Autodesk Inventor part; units mm, degrees
(part 2 of 3)
  circle A470 centre (-52.8488, 38.1375) radius 0.851
  circle A471 centre (-42.6888, 38.1375) radius 0.851
  circle A472 centre (-38.2437, 19.0875) radius 1.994
  circle A473 centre (-43.3237, 19.0875) radius 0.851
  circle A474 centre (-33.1638, 19.0875) radius 0.851
  circle A475 centre (-33.4813, 0.0375) radius 1.994
  circle A476 centre (-38.5613, 0.0375) radius 0.851
  circle A477 centre (-28.4013, 0.0375) radius 0.851
  circle A478 centre (-23.9563, -19.0125) radius 1.994
  circle A479 centre (-29.0362, -19.0125) radius 0.851
  circle A480 centre (-18.8762, -19.0125) radius 0.851
  circle A481 centre (-135.875, 0.0375) radius 1.994
  circle A482 centre (-140.955, 0.0375) radius 0.851
  circle A483 centre (-130.795, 0.0375) radius 0.851
  circle A484 centre (-28.7188, 38.1375) radius 1.994
  circle A485 centre (-33.7987, 38.1375) radius 0.851
  circle A486 centre (-23.6388, 38.1375) radius 0.851
  circle A487 centre (-19.1938, 19.0875) radius 1.994
  circle A488 centre (-24.2737, 19.0875) radius 0.851
  circle A489 centre (-14.1137, 19.0875) radius 0.851
  circle A490 centre (-14.4313, 0.0375) radius 1.994
  circle A491 centre (-19.5113, 0.0375) radius 0.851
  circle A492 centre (-9.3513, 0.0375) radius 0.851
  circle A493 centre (-4.9062, -19.0125) radius 1.994
  circle A494 centre (-9.9863, -19.0125) radius 0.851
  circle A495 centre (0.1737, -19.0125) radius 0.851
  circle A496 centre (-21.575, -38.0625) radius 1.994
  circle A497 centre (-26.655, -38.0625) radius 0.851
  circle A498 centre (-16.495, -38.0625) radius 0.851
  circle A499 centre (-71.613, -31.0775) radius 1.524
  circle A500 centre (28.463, -31.0775) radius 1.524
  circle A501 centre (-71.613, -46.3175) radius 1.994
  circle A502 centre (28.463, -46.3175) radius 1.994
  circle A503 centre (-9.6687, 38.1375) radius 1.994
  circle A504 centre (-14.7487, 38.1375) radius 0.851
  circle A505 centre (-4.5888, 38.1375) radius 0.851
  circle A506 centre (-0.1437, 19.0875) radius 1.994
  circle A507 centre (-5.2238, 19.0875) radius 0.851
  circle A508 centre (4.9363, 19.0875) radius 0.851
  circle A509 centre (4.6188, 0.0375) radius 1.994
  circle A510 centre (-0.4612, 0.0375) radius 0.851
  circle A511 centre (9.6988, 0.0375) radius 0.851
  circle A512 centre (14.1438, -19.0125) radius 1.994
  circle A513 centre (9.0638, -19.0125) radius 0.851
  circle A514 centre (19.2237, -19.0125) radius 0.851
  circle A515 centre (-131.1125, -19.0125) radius 1.994
  circle A516 centre (-136.1925, -19.0125) radius 0.851
  circle A517 centre (-126.0325, -19.0125) radius 0.851
  circle A518 centre (-143.0505, -12.0275) radius 1.524
  circle A519 centre (-119.1745, -12.0275) radius 1.524
  circle A520 centre (-143.0505, -27.2675) radius 1.994
  circle A521 centre (-119.1745, -27.2675) radius 1.994
  circle A522 centre (9.3812, 38.1375) radius 1.994
  circle A523 centre (4.3012, 38.1375) radius 0.851
  circle A524 centre (14.4613, 38.1375) radius 0.851
  circle A525 centre (18.9062, 19.0875) radius 1.994
  circle A526 centre (13.8262, 19.0875) radius 0.851
  circle A527 centre (23.9862, 19.0875) radius 0.851
  circle A528 centre (23.6687, 0.0375) radius 1.994
  circle A529 centre (18.5888, 0.0375) radius 0.851
  circle A530 centre (28.7488, 0.0375) radius 0.851
  circle A531 centre (33.1938, -19.0125) radius 1.994
  circle A532 centre (28.1137, -19.0125) radius 0.851
  circle A533 centre (38.2737, -19.0125) radius 0.851
  circle A534 centre (28.4313, 38.1375) radius 1.994
  circle A535 centre (23.3513, 38.1375) radius 0.851
  circle A536 centre (33.5112, 38.1375) radius 0.851
  circle A537 centre (37.9562, 19.0875) radius 1.994
  circle A538 centre (32.8762, 19.0875) radius 0.851
  circle A539 centre (43.0363, 19.0875) radius 0.851
  circle A540 centre (42.7188, 0.0375) radius 1.994
  circle A541 centre (37.6388, 0.0375) radius 0.851
  circle A542 centre (47.7987, 0.0375) radius 0.851
  circle A543 centre (52.2438, -19.0125) radius 1.994
  circle A544 centre (47.1638, -19.0125) radius 0.851
  circle A545 centre (57.3238, -19.0125) radius 0.851
  circle A546 centre (-140.6375, -38.0625) radius 1.994
  circle A547 centre (-145.7175, -38.0625) radius 0.851
  circle A548 centre (-135.5575, -38.0625) radius 0.851
  circle A549 centre (47.4813, 38.1375) radius 1.994
  circle A550 centre (42.4012, 38.1375) radius 0.851
  circle A551 centre (52.5613, 38.1375) radius 0.851
  circle A552 centre (57.0063, 19.0875) radius 1.994
  circle A553 centre (51.9263, 19.0875) radius 0.851
  circle A554 centre (62.0863, 19.0875) radius 0.851
  circle A555 centre (61.7687, 0.0375) radius 1.994
  circle A556 centre (56.6887, 0.0375) radius 0.851
  circle A557 centre (66.8487, 0.0375) radius 0.851
  circle A558 centre (71.2938, -19.0125) radius 1.994
  circle A559 centre (66.2138, -19.0125) radius 0.851
  circle A560 centre (76.3738, -19.0125) radius 0.851
  circle A561 centre (47.4813, -38.0625) radius 1.994
  circle A562 centre (42.4012, -38.0625) radius 0.851
  circle A563 centre (52.5613, -38.0625) radius 0.851
  circle A564 centre (66.5312, 38.1375) radius 1.994
  circle A565 centre (61.4513, 38.1375) radius 0.851
  circle A566 centre (71.6112, 38.1375) radius 0.851
  circle A567 centre (76.0563, 19.0875) radius 1.994
  circle A568 centre (70.9762, 19.0875) radius 0.851
  circle A569 centre (81.1363, 19.0875) radius 0.851
  circle A570 centre (80.8187, 0.0375) radius 1.994
  circle A571 centre (75.7387, 0.0375) radius 0.851
  circle A572 centre (85.8988, 0.0375) radius 0.851
  circle A573 centre (97.4875, -19.0125) radius 1.994
  circle A574 centre (92.4075, -19.0125) radius 0.851
  circle A575 centre (102.5675, -19.0125) radius 0.851
  circle A576 centre (-123.9688, 38.1375) radius 1.994
  circle A577 centre (-129.0488, 38.1375) radius 0.851
  circle A578 centre (-118.8888, 38.1375) radius 0.851
  circle A579 centre (66.5312, -38.0625) radius 1.994
  circle A580 centre (61.4513, -38.0625) radius 0.851
  circle A581 centre (71.6112, -38.0625) radius 0.851
  circle A582 centre (85.5813, 38.1375) radius 1.994
  circle A583 centre (80.5012, 38.1375) radius 0.851
  circle A584 centre (90.6612, 38.1375) radius 0.851
  circle A585 centre (95.1063, 19.0875) radius 1.994
  circle A586 centre (90.0263, 19.0875) radius 0.851
  circle A587 centre (100.1863, 19.0875) radius 0.851
  circle A588 centre (111.775, 0.0375) radius 1.994
  circle A589 centre (106.695, 0.0375) radius 0.851
  circle A590 centre (116.855, 0.0375) radius 0.851
  circle A591 centre (99.837, 7.0225) radius 1.524
  circle A592 centre (123.713, 7.0225) radius 1.524
  circle A593 centre (99.837, -8.2175) radius 1.994
  circle A594 centre (123.713, -8.2175) radius 1.994
  circle A595 centre (123.6813, -19.0125) radius 1.994
  circle A596 centre (118.6012, -19.0125) radius 0.851
  circle A597 centre (128.7612, -19.0125) radius 0.851
  circle A598 centre (85.5813, -38.0625) radius 1.994
  circle A599 centre (80.5012, -38.0625) radius 0.851
  circle A600 centre (90.6612, -38.0625) radius 0.851
  circle A601 centre (114.1562, 38.1375) radius 1.994
  circle A602 centre (109.0763, 38.1375) radius 0.851
  circle A603 centre (119.2363, 38.1375) radius 0.851
  circle A604 centre (102.2183, 45.1225) radius 1.524
  circle A605 centre (126.0943, 45.1225) radius 1.524
  circle A606 centre (102.2183, 29.8825) radius 1.994
  circle A607 centre (126.0943, 29.8825) radius 1.994
  circle A608 centre (118.9188, 19.0875) radius 1.994
  circle A609 centre (113.8388, 19.0875) radius 0.851
  circle A610 centre (123.9988, 19.0875) radius 0.851
  circle A611 centre (142.7312, 0.0375) radius 1.994
  circle A612 centre (137.6513, 0.0375) radius 0.851
  circle A613 centre (147.8113, 0.0375) radius 0.851
  circle A614 centre (142.7312, -19.0125) radius 1.994
  circle A615 centre (137.6513, -19.0125) radius 0.851
  circle A616 centre (147.8113, -19.0125) radius 0.851
  circle A617 centre (-114.4438, 19.0875) radius 1.994
  circle A618 centre (-119.5238, 19.0875) radius 0.851
  circle A619 centre (-109.3637, 19.0875) radius 0.851
  circle A620 centre (123.6813, -38.0625) radius 1.994
  circle A621 centre (118.6012, -38.0625) radius 0.851
  circle A622 centre (128.7612, -38.0625) radius 0.851
  circle A623 centre (142.7312, 38.1375) radius 1.994
  circle A624 centre (137.6513, 38.1375) radius 0.851
  circle A625 centre (147.8113, 38.1375) radius 0.851
  circle A626 centre (142.7312, 19.0875) radius 1.994
  circle A627 centre (137.6513, 19.0875) radius 0.851
  circle A628 centre (147.8113, 19.0875) radius 0.851
  circle A629 centre (104.6312, -38.0625) radius 1.994
  circle A630 centre (99.5513, -38.0625) radius 0.851
  circle A631 centre (109.7113, -38.0625) radius 0.851
  circle A632 centre (142.7312, -38.0625) radius 1.994
  circle A633 centre (137.6513, -38.0625) radius 0.851
  circle A634 centre (147.8113, -38.0625) radius 0.851
  circle A635 centre (-109.6813, 0.0375) radius 1.994
  circle A636 centre (-114.7613, 0.0375) radius 0.851
  circle A637 centre (-104.6012, 0.0375) radius 0.851
  circle A638 centre (-100.1562, -19.0125) radius 1.994
  circle A639 centre (-105.2363, -19.0125) radius 0.851
  circle A640 centre (-95.0763, -19.0125) radius 0.851
  line L292 (-141.5265, 49.25) -> (-141.5265, 61.95)
  line L293 (-153.375, 43.2168) -> (-159.725, 43.2168)
  line L294 (153.375, -39.5103) -> (159.725, -39.5103)
  line L295 (148.216, -49.25) -> (148.216, -61.95)
  line L296 (-159.725, 61.95) -> (159.725, 61.95)
  line L297 (159.725, 61.95) -> (159.725, -61.95)
  line L298 (159.725, -61.95) -> (-159.725, -61.95)
  line L299 (-159.725, -61.95) -> (-159.725, 61.95)
  line L300 (-159.725, 61.95) -> (-159.725, 87.35)
  line L301 (-159.725, 87.35) -> (159.725, 87.35)
  line L302 (159.725, 87.35) -> (159.725, 61.95)
  line L303 (-159.725, 87.35) -> (-159.725, 93.7)
  line L304 (-153.375, 100.05) -> (153.375, 100.05)
  line L305 (159.725, 93.7) -> (159.725, 87.35)
  line L306 (-159.725, -61.95) -> (-159.725, -74.65)
  line L307 (-159.725, -74.65) -> (159.725, -74.65)
  line L308 (159.725, -74.65) -> (159.725, -61.95)
  line L309 (-159.725, -74.65) -> (-159.725, -81)
  line L310 (-153.375, -87.35) -> (153.375, -87.35)
  line L311 (159.725, -81) -> (159.725, -74.65)
  arc A641 (-153.375, 100.05) -> (-159.725, 93.7) centre (-153.375, 93.7) ccw
  arc A642 (159.725, 93.7) -> (153.375, 100.05) centre (153.375, 93.7) ccw
  arc A643 (153.375, -87.35) -> (159.725, -81) centre (153.375, -81) ccw
  arc A644 (-159.725, -81) -> (-153.375, -87.35) centre (-153.375, -81) ccw
  arc A645 (-150.0419, 31.4192) -> (-149.7371, 31.1144) centre (-149.7371, 31.4192) ccw
  arc A646 (-149.7371, 45.1606) -> (-150.0419, 44.8558) centre (-149.7371, 44.8558) ccw
  line L312 (-150.0419, 44.8558) -> (-150.0419, 31.4192)
  arc A647 (-135.9956, 44.8558) -> (-136.3005, 45.1606) centre (-136.3005, 44.8558) ccw
  line L313 (-135.9956, 31.4192) -> (-135.9956, 44.8558)
  line L314 (-149.7371, 31.1144) -> (-136.3005, 31.1144)
  line L315 (-150.0419, 31.1144) -> (-135.9956, 45.1606) construction
  line L316 (-135.9956, 31.1144) -> (-150.0419, 45.1606) construction
  arc A648 (-136.3005, 31.1144) -> (-135.9956, 31.4192) centre (-136.3005, 31.4192) ccw
  line L317 (-136.3005, 45.1606) -> (-149.7371, 45.1606)
  arc A649 (-130.9918, 31.4192) -> (-130.687, 31.1144) centre (-130.687, 31.4192) ccw
  arc A650 (-130.687, 45.1606) -> (-130.9918, 44.8558) centre (-130.687, 44.8558) ccw
  line L318 (-130.9918, 44.8558) -> (-130.9918, 31.4192)
  arc A651 (-116.9456, 44.8558) -> (-117.2505, 45.1606) centre (-117.2505, 44.8558) ccw
  line L319 (-116.9456, 31.4192) -> (-116.9456, 44.8558)
  line L320 (-130.687, 31.1144) -> (-117.2505, 31.1144)
  line L321 (-130.9918, 31.1144) -> (-116.9456, 45.1606) construction
  line L322 (-116.9456, 31.1144) -> (-130.9918, 45.1606) construction
  arc A652 (-117.2505, 31.1144) -> (-116.9456, 31.4192) centre (-117.2505, 31.4192) ccw
  line L323 (-117.2505, 45.1606) -> (-130.687, 45.1606)
  arc A653 (-145.2793, 12.3692) -> (-144.9745, 12.0644) centre (-144.9745, 12.3692) ccw
  arc A654 (-144.9745, 26.1106) -> (-145.2793, 25.8058) centre (-144.9745, 25.8058) ccw
  line L324 (-145.2793, 25.8058) -> (-145.2793, 12.3692)
  arc A655 (-131.2331, 25.8058) -> (-131.5379, 26.1106) centre (-131.5379, 25.8058) ccw
  line L325 (-131.2331, 12.3692) -> (-131.2331, 25.8058)
  line L326 (-144.9745, 12.0644) -> (-131.5379, 12.0644)
  line L327 (-145.2793, 12.0644) -> (-131.2331, 26.1106) construction
  line L328 (-131.2331, 12.0644) -> (-145.2793, 26.1106) construction
  arc A656 (-131.5379, 12.0644) -> (-131.2331, 12.3692) centre (-131.5379, 12.3692) ccw
  line L329 (-131.5379, 26.1106) -> (-144.9745, 26.1106)
  arc A657 (-121.4668, 12.3692) -> (-121.1621, 12.0644) centre (-121.1621, 12.3692) ccw
  arc A658 (-121.1621, 26.1106) -> (-121.4668, 25.8058) centre (-121.1621, 25.8058) ccw
  line L330 (-121.4668, 25.8058) -> (-121.4668, 12.3692)
  arc A659 (-107.4206, 25.8058) -> (-107.7255, 26.1106) centre (-107.7255, 25.8058) ccw
  line L331 (-107.4206, 12.3692) -> (-107.4206, 25.8058)
  line L332 (-121.1621, 12.0644) -> (-107.7255, 12.0644)
  line L333 (-121.4668, 12.0644) -> (-107.4206, 26.1106) construction
  line L334 (-107.4206, 12.0644) -> (-121.4668, 26.1106) construction
  arc A660 (-107.7255, 12.0644) -> (-107.4206, 12.3692) centre (-107.7255, 12.3692) ccw
  line L335 (-107.7255, 26.1106) -> (-121.1621, 26.1106)
  arc A661 (-142.8981, -6.6808) -> (-142.5933, -6.9856) centre (-142.5933, -6.6808) ccw
  arc A662 (-142.5933, 7.0606) -> (-142.8981, 6.7558) centre (-142.5933, 6.7558) ccw
  line L336 (-142.8981, 6.7558) -> (-142.8981, -6.6808)
  arc A663 (-128.8519, 6.7558) -> (-129.1567, 7.0606) centre (-129.1567, 6.7558) ccw
  line L337 (-128.8519, -6.6808) -> (-128.8519, 6.7558)
  line L338 (-142.5933, -6.9856) -> (-129.1567, -6.9856)
  line L339 (-142.8981, -6.9856) -> (-128.8519, 7.0606) construction
  line L340 (-128.8519, -6.9856) -> (-142.8981, 7.0606) construction
  arc A664 (-129.1567, -6.9856) -> (-128.8519, -6.6808) centre (-129.1567, -6.6808) ccw
  line L341 (-129.1567, 7.0606) -> (-142.5933, 7.0606)
  arc A665 (-116.7043, -6.6808) -> (-116.3996, -6.9856) centre (-116.3996, -6.6808) ccw
  arc A666 (-116.3996, 7.0606) -> (-116.7043, 6.7558) centre (-116.3996, 6.7558) ccw
  line L342 (-116.7043, 6.7558) -> (-116.7043, -6.6808)
  arc A667 (-102.6581, 6.7558) -> (-102.963, 7.0606) centre (-102.963, 6.7558) ccw
  line L343 (-102.6581, -6.6808) -> (-102.6581, 6.7558)
  line L344 (-116.3996, -6.9856) -> (-102.963, -6.9856)
  line L345 (-116.7043, -6.9856) -> (-102.6581, 7.0606) construction
  line L346 (-102.6581, -6.9856) -> (-116.7043, 7.0606) construction
  arc A668 (-102.963, -6.9856) -> (-102.6581, -6.6808) centre (-102.963, -6.6808) ccw
  line L347 (-102.963, 7.0606) -> (-116.3996, 7.0606)
  arc A669 (-107.1793, -25.7308) -> (-106.8745, -26.0356) centre (-106.8745, -25.7308) ccw
  arc A670 (-106.8745, -11.9894) -> (-107.1793, -12.2942) centre (-106.8745, -12.2942) ccw
  line L348 (-107.1793, -12.2942) -> (-107.1793, -25.7308)
  arc A671 (-93.1331, -12.2942) -> (-93.438, -11.9894) centre (-93.438, -12.2942) ccw
  line L349 (-93.1331, -25.7308) -> (-93.1331, -12.2942)
  line L350 (-106.8745, -26.0356) -> (-93.438, -26.0356)
  line L351 (-107.1793, -26.0356) -> (-93.1331, -11.9894) construction
  line L352 (-93.1331, -26.0356) -> (-107.1793, -11.9894) construction
  arc A672 (-93.438, -26.0356) -> (-93.1331, -25.7308) centre (-93.438, -25.7308) ccw
  line L353 (-93.438, -11.9894) -> (-106.8745, -11.9894)
  arc A673 (-147.6606, -44.7808) -> (-147.3558, -45.0856) centre (-147.3558, -44.7808) ccw
  arc A674 (-147.3558, -31.0394) -> (-147.6606, -31.3442) centre (-147.3558, -31.3442) ccw
  line L354 (-147.6606, -31.3442) -> (-147.6606, -44.7808)
  arc A675 (-133.6144, -31.3442) -> (-133.9192, -31.0394) centre (-133.9192, -31.3442) ccw
  line L355 (-133.6144, -44.7808) -> (-133.6144, -31.3442)
  line L356 (-147.3558, -45.0856) -> (-133.9192, -45.0856)
  line L357 (-147.6606, -45.0856) -> (-133.6144, -31.0394) construction
  line L358 (-133.6144, -45.0856) -> (-147.6606, -31.0394) construction
  arc A676 (-133.9192, -45.0856) -> (-133.6144, -44.7808) centre (-133.9192, -44.7808) ccw
  line L359 (-133.9192, -31.0394) -> (-147.3558, -31.0394)
  arc A677 (-123.8481, -44.7808) -> (-123.5433, -45.0856) centre (-123.5433, -44.7808) ccw
  arc A678 (-123.5433, -31.0394) -> (-123.8481, -31.3442) centre (-123.5433, -31.3442) ccw
  line L360 (-123.8481, -31.3442) -> (-123.8481, -44.7808)
  arc A679 (-109.8019, -31.3442) -> (-110.1067, -31.0394) centre (-110.1067, -31.3442) ccw
  line L361 (-109.8019, -44.7808) -> (-109.8019, -31.3442)
  line L362 (-123.5433, -45.0856) -> (-110.1067, -45.0856)
  line L363 (-123.8481, -45.0856) -> (-109.8019, -31.0394) construction
  line L364 (-109.8019, -45.0856) -> (-123.8481, -31.0394) construction
  arc A680 (-110.1067, -45.0856) -> (-109.8019, -44.7808) centre (-110.1067, -44.7808) ccw
  line L365 (-110.1067, -31.0394) -> (-123.5433, -31.0394)
  arc A681 (-100.0356, -44.7808) -> (-99.7308, -45.0856) centre (-99.7308, -44.7808) ccw
  arc A682 (-99.7308, -31.0394) -> (-100.0356, -31.3442) centre (-99.7308, -31.3442) ccw
  line L366 (-100.0356, -31.3442) -> (-100.0356, -44.7808)
  arc A683 (-85.9894, -31.3442) -> (-86.2942, -31.0394) centre (-86.2942, -31.3442) ccw
  line L367 (-85.9894, -44.7808) -> (-85.9894, -31.3442)
  line L368 (-99.7308, -45.0856) -> (-86.2942, -45.0856)
  line L369 (-100.0356, -45.0856) -> (-85.9894, -31.0394) construction
  line L370 (-85.9894, -45.0856) -> (-100.0356, -31.0394) construction
  arc A684 (-86.2942, -45.0856) -> (-85.9894, -44.7808) centre (-86.2942, -44.7808) ccw
  line L371 (-86.2942, -31.0394) -> (-99.7308, -31.0394)
  arc A685 (-88.1293, -25.7308) -> (-87.8246, -26.0356) centre (-87.8246, -25.7308) ccw
  arc A686 (-87.8246, -11.9894) -> (-88.1293, -12.2942) centre (-87.8246, -12.2942) ccw
  line L372 (-88.1293, -12.2942) -> (-88.1293, -25.7308)
  arc A687 (-74.0831, -12.2942) -> (-74.388, -11.9894) centre (-74.388, -12.2942) ccw
  line L373 (-74.0831, -25.7308) -> (-74.0831, -12.2942)
  line L374 (-87.8246, -26.0356) -> (-74.388, -26.0356)
  line L375 (-88.1293, -26.0356) -> (-74.0831, -11.9894) construction
  line L376 (-74.0831, -26.0356) -> (-88.1293, -11.9894) construction
  arc A688 (-74.388, -26.0356) -> (-74.0831, -25.7308) centre (-74.388, -25.7308) ccw
  line L377 (-74.388, -11.9894) -> (-87.8246, -11.9894)
  arc A689 (-97.6543, -6.6808) -> (-97.3495, -6.9856) centre (-97.3495, -6.6808) ccw
  arc A690 (-97.3495, 7.0606) -> (-97.6543, 6.7558) centre (-97.3495, 6.7558) ccw
  line L378 (-97.6543, 6.7558) -> (-97.6543, -6.6808)
  arc A691 (-83.6081, 6.7558) -> (-83.9129, 7.0606) centre (-83.9129, 6.7558) ccw
  line L379 (-83.6081, -6.6808) -> (-83.6081, 6.7558)
  line L380 (-97.3495, -6.9856) -> (-83.9129, -6.9856)
  line L381 (-97.6543, -6.9856) -> (-83.6081, 7.0606) construction
  line L382 (-83.6081, -6.9856) -> (-97.6543, 7.0606) construction
  arc A692 (-83.9129, -6.9856) -> (-83.6081, -6.6808) centre (-83.9129, -6.6808) ccw
  line L383 (-83.9129, 7.0606) -> (-97.3495, 7.0606)
  arc A693 (-102.4168, 12.3692) -> (-102.112, 12.0644) centre (-102.112, 12.3692) ccw
  arc A694 (-102.112, 26.1106) -> (-102.4168, 25.8058) centre (-102.112, 25.8058) ccw
  line L384 (-102.4168, 25.8058) -> (-102.4168, 12.3692)
  arc A695 (-88.3706, 25.8058) -> (-88.6754, 26.1106) centre (-88.6754, 25.8058) ccw
  line L385 (-88.3706, 12.3692) -> (-88.3706, 25.8058)
  line L386 (-102.112, 12.0644) -> (-88.6754, 12.0644)
  line L387 (-102.4168, 12.0644) -> (-88.3706, 26.1106) construction
  line L388 (-88.3706, 12.0644) -> (-102.4168, 26.1106) construction
  arc A696 (-88.6754, 12.0644) -> (-88.3706, 12.3692) centre (-88.6754, 12.3692) ccw
  line L389 (-88.6754, 26.1106) -> (-102.112, 26.1106)
  arc A697 (-111.9418, 31.4192) -> (-111.6371, 31.1144) centre (-111.6371, 31.4192) ccw
  arc A698 (-111.6371, 45.1606) -> (-111.9418, 44.8558) centre (-111.6371, 44.8558) ccw
  line L390 (-111.9418, 44.8558) -> (-111.9418, 31.4192)
  arc A699 (-97.8956, 44.8558) -> (-98.2005, 45.1606) centre (-98.2005, 44.8558) ccw
  line L391 (-97.8956, 31.4192) -> (-97.8956, 44.8558)
  line L392 (-111.6371, 31.1144) -> (-98.2005, 31.1144)
  line L393 (-111.9418, 31.1144) -> (-97.8956, 45.1606) construction
  line L394 (-97.8956, 31.1144) -> (-111.9418, 45.1606) construction
  arc A700 (-98.2005, 31.1144) -> (-97.8956, 31.4192) centre (-98.2005, 31.4192) ccw
  line L395 (-98.2005, 45.1606) -> (-111.6371, 45.1606)
  arc A701 (-92.8918, 31.4192) -> (-92.5871, 31.1144) centre (-92.5871, 31.4192) ccw
  arc A702 (-92.5871, 45.1606) -> (-92.8918, 44.8558) centre (-92.5871, 44.8558) ccw
  line L396 (-92.8918, 44.8558) -> (-92.8918, 31.4192)
  arc A703 (-78.8456, 44.8558) -> (-79.1505, 45.1606) centre (-79.1505, 44.8558) ccw
  line L397 (-78.8456, 31.4192) -> (-78.8456, 44.8558)
  line L398 (-92.5871, 31.1144) -> (-79.1505, 31.1144)
  line L399 (-92.8918, 31.1144) -> (-78.8456, 45.1606) construction
  line L400 (-78.8456, 31.1144) -> (-92.8918, 45.1606) construction
  arc A704 (-79.1505, 31.1144) -> (-78.8456, 31.4192) centre (-79.1505, 31.4192) ccw
  line L401 (-79.1505, 45.1606) -> (-92.5871, 45.1606)
  arc A705 (-73.8418, 31.4192) -> (-73.537, 31.1144) centre (-73.537, 31.4192) ccw
  arc A706 (-73.537, 45.1606) -> (-73.8418, 44.8558) centre (-73.537, 44.8558) ccw
  line L402 (-73.8418, 44.8558) -> (-73.8418, 31.4192)
  arc A707 (-59.7956, 44.8558) -> (-60.1004, 45.1606) centre (-60.1004, 44.8558) ccw
  line L403 (-59.7956, 31.4192) -> (-59.7956, 44.8558)
  line L404 (-73.537, 31.1144) -> (-60.1004, 31.1144)
  line L405 (-73.8418, 31.1144) -> (-59.7956, 45.1606) construction
  line L406 (-59.7956, 31.1144) -> (-73.8418, 45.1606) construction
  arc A708 (-60.1004, 31.1144) -> (-59.7956, 31.4192) centre (-60.1004, 31.4192) ccw
  line L407 (-60.1004, 45.1606) -> (-73.537, 45.1606)
  arc A709 (-83.3668, 12.3692) -> (-83.062, 12.0644) centre (-83.062, 12.3692) ccw
  arc A710 (-83.062, 26.1106) -> (-83.3668, 25.8058) centre (-83.062, 25.8058) ccw
  line L408 (-83.3668, 25.8058) -> (-83.3668, 12.3692)
  arc A711 (-69.3206, 25.8058) -> (-69.6255, 26.1106) centre (-69.6255, 25.8058) ccw
  line L409 (-69.3206, 12.3692) -> (-69.3206, 25.8058)
  line L410 (-83.062, 12.0644) -> (-69.6255, 12.0644)
  line L411 (-83.3668, 12.0644) -> (-69.3206, 26.1106) construction
  line L412 (-69.3206, 12.0644) -> (-83.3668, 26.1106) construction
  arc A712 (-69.6255, 12.0644) -> (-69.3206, 12.3692) centre (-69.6255, 12.3692) ccw
  line L413 (-69.6255, 26.1106) -> (-83.062, 26.1106)
  arc A713 (-64.3168, 12.3692) -> (-64.0121, 12.0644) centre (-64.0121, 12.3692) ccw
  arc A714 (-64.0121, 26.1106) -> (-64.3168, 25.8058) centre (-64.0121, 25.8058) ccw
  line L414 (-64.3168, 25.8058) -> (-64.3168, 12.3692)
  arc A715 (-50.2706, 25.8058) -> (-50.5755, 26.1106) centre (-50.5755, 25.8058) ccw
  line L415 (-50.2706, 12.3692) -> (-50.2706, 25.8058)
  line L416 (-64.0121, 12.0644) -> (-50.5755, 12.0644)
  line L417 (-64.3168, 12.0644) -> (-50.2706, 26.1106) construction
  line L418 (-50.2706, 12.0644) -> (-64.3168, 26.1106) construction
  arc A716 (-50.5755, 12.0644) -> (-50.2706, 12.3692) centre (-50.5755, 12.3692) ccw
  line L419 (-50.5755, 26.1106) -> (-64.0121, 26.1106)
  arc A717 (-78.6043, -6.6808) -> (-78.2995, -6.9856) centre (-78.2995, -6.6808) ccw
  arc A718 (-78.2995, 7.0606) -> (-78.6043, 6.7558) centre (-78.2995, 6.7558) ccw
  line L420 (-78.6043, 6.7558) -> (-78.6043, -6.6808)
  arc A719 (-64.5581, 6.7558) -> (-64.8629, 7.0606) centre (-64.8629, 6.7558) ccw
  line L421 (-64.5581, -6.6808) -> (-64.5581, 6.7558)
  line L422 (-78.2995, -6.9856) -> (-64.8629, -6.9856)
  line L423 (-78.6043, -6.9856) -> (-64.5581, 7.0606) construction
  line L424 (-64.5581, -6.9856) -> (-78.6043, 7.0606) construction
  arc A720 (-64.8629, -6.9856) -> (-64.5581, -6.6808) centre (-64.8629, -6.6808) ccw
  line L425 (-64.8629, 7.0606) -> (-78.2995, 7.0606)
  arc A721 (-59.5543, -6.6808) -> (-59.2496, -6.9856) centre (-59.2496, -6.6808) ccw
  arc A722 (-59.2496, 7.0606) -> (-59.5543, 6.7558) centre (-59.2496, 6.7558) ccw
  line L426 (-59.5543, 6.7558) -> (-59.5543, -6.6808)
  arc A723 (-45.5081, 6.7558) -> (-45.813, 7.0606) centre (-45.813, 6.7558) ccw
  line L427 (-45.5081, -6.6808) -> (-45.5081, 6.7558)
  line L428 (-59.2496, -6.9856) -> (-45.813, -6.9856)
  line L429 (-59.5543, -6.9856) -> (-45.5081, 7.0606) construction
  line L430 (-45.5081, -6.9856) -> (-59.5543, 7.0606) construction
  arc A724 (-45.813, -6.9856) -> (-45.5081, -6.6808) centre (-45.813, -6.6808) ccw
  line L431 (-45.813, 7.0606) -> (-59.2496, 7.0606)
  arc A725 (-69.0793, -25.7308) -> (-68.7746, -26.0356) centre (-68.7746, -25.7308) ccw
  arc A726 (-68.7746, -11.9894) -> (-69.0793, -12.2942) centre (-68.7746, -12.2942) ccw
  line L432 (-69.0793, -12.2942) -> (-69.0793, -25.7308)
  arc A727 (-55.0331, -12.2942) -> (-55.338, -11.9894) centre (-55.338, -12.2942) ccw
  line L433 (-55.0331, -25.7308) -> (-55.0331, -12.2942)
  line L434 (-68.7746, -26.0356) -> (-55.338, -26.0356)
  line L435 (-69.0793, -26.0356) -> (-55.0331, -11.9894) construction
  line L436 (-55.0331, -26.0356) -> (-69.0793, -11.9894) construction
  arc A728 (-55.338, -26.0356) -> (-55.0331, -25.7308) centre (-55.338, -25.7308) ccw
  line L437 (-55.338, -11.9894) -> (-68.7746, -11.9894)
  arc A729 (-50.0293, -25.7308) -> (-49.7246, -26.0356) centre (-49.7246, -25.7308) ccw
  arc A730 (-49.7246, -11.9894) -> (-50.0293, -12.2942) centre (-49.7246, -12.2942) ccw
  line L438 (-50.0293, -12.2942) -> (-50.0293, -25.7308)
  arc A731 (-35.9831, -12.2942) -> (-36.288, -11.9894) centre (-36.288, -12.2942) ccw
  line L439 (-35.9831, -25.7308) -> (-35.9831, -12.2942)
  line L440 (-49.7246, -26.0356) -> (-36.288, -26.0356)
  line L441 (-50.0293, -26.0356) -> (-35.9831, -11.9894) construction
  line L442 (-35.9831, -26.0356) -> (-50.0293, -11.9894) construction
  arc A732 (-36.288, -26.0356) -> (-35.9831, -25.7308) centre (-36.288, -25.7308) ccw
  line L443 (-36.288, -11.9894) -> (-49.7246, -11.9894)
  arc A733 (-54.7918, 31.4192) -> (-54.4871, 31.1144) centre (-54.4871, 31.4192) ccw
  arc A734 (-54.4871, 45.1606) -> (-54.7918, 44.8558) centre (-54.4871, 44.8558) ccw
  line L444 (-54.7918, 44.8558) -> (-54.7918, 31.4192)
  arc A735 (-40.7456, 44.8558) -> (-41.0505, 45.1606) centre (-41.0505, 44.8558) ccw
  line L445 (-40.7456, 31.4192) -> (-40.7456, 44.8558)
  line L446 (-54.4871, 31.1144) -> (-41.0505, 31.1144)
  line L447 (-54.7918, 31.1144) -> (-40.7456, 45.1606) construction
  line L448 (-40.7456, 31.1144) -> (-54.7918, 45.1606) construction
  arc A736 (-41.0505, 31.1144) -> (-40.7456, 31.4192) centre (-41.0505, 31.4192) ccw
  line L449 (-41.0505, 45.1606) -> (-54.4871, 45.1606)
  arc A737 (-45.2668, 12.3692) -> (-44.962, 12.0644) centre (-44.962, 12.3692) ccw
  arc A738 (-44.962, 26.1106) -> (-45.2668, 25.8058) centre (-44.962, 25.8058) ccw
  line L450 (-45.2668, 25.8058) -> (-45.2668, 12.3692)
  arc A739 (-31.2206, 25.8058) -> (-31.5254, 26.1106) centre (-31.5254, 25.8058) ccw
  line L451 (-31.2206, 12.3692) -> (-31.2206, 25.8058)
  line L452 (-44.962, 12.0644) -> (-31.5254, 12.0644)
  line L453 (-45.2668, 12.0644) -> (-31.2206, 26.1106) construction
  line L454 (-31.2206, 12.0644) -> (-45.2668, 26.1106) construction
  arc A740 (-31.5254, 12.0644) -> (-31.2206, 12.3692) centre (-31.5254, 12.3692) ccw
  line L455 (-31.5254, 26.1106) -> (-44.962, 26.1106)
  arc A741 (-40.5043, -6.6808) -> (-40.1995, -6.9856) centre (-40.1995, -6.6808) ccw
  arc A742 (-40.1995, 7.0606) -> (-40.5043, 6.7558) centre (-40.1995, 6.7558) ccw
  line L456 (-40.5043, 6.7558) -> (-40.5043, -6.6808)
  arc A743 (-26.4581, 6.7558) -> (-26.7629, 7.0606) centre (-26.7629, 6.7558) ccw
  line L457 (-26.4581, -6.6808) -> (-26.4581, 6.7558)
  line L458 (-40.1995, -6.9856) -> (-26.7629, -6.9856)
  line L459 (-40.5043, -6.9856) -> (-26.4581, 7.0606) construction
  line L460 (-26.4581, -6.9856) -> (-40.5043, 7.0606) construction
  arc A744 (-26.7629, -6.9856) -> (-26.4581, -6.6808) centre (-26.7629, -6.6808) ccw
  line L461 (-26.7629, 7.0606) -> (-40.1995, 7.0606)
  arc A745 (-30.9793, -25.7308) -> (-30.6745, -26.0356) centre (-30.6745, -25.7308) ccw
  arc A746 (-30.6745, -11.9894) -> (-30.9793, -12.2942) centre (-30.6745, -12.2942) ccw
  line L462 (-30.9793, -12.2942) -> (-30.9793, -25.7308)
  arc A747 (-16.9331, -12.2942) -> (-17.2379, -11.9894) centre (-17.2379, -12.2942) ccw
  line L463 (-16.9331, -25.7308) -> (-16.9331, -12.2942)
  line L464 (-30.6745, -26.0356) -> (-17.2379, -26.0356)
  line L465 (-30.9793, -26.0356) -> (-16.9331, -11.9894) construction
  line L466 (-16.9331, -26.0356) -> (-30.9793, -11.9894) construction
  arc A748 (-17.2379, -26.0356) -> (-16.9331, -25.7308) centre (-17.2379, -25.7308) ccw
  line L467 (-17.2379, -11.9894) -> (-30.6745, -11.9894)
  arc A749 (-35.7418, 31.4192) -> (-35.437, 31.1144) centre (-35.437, 31.4192) ccw
  arc A750 (-35.437, 45.1606) -> (-35.7418, 44.8558) centre (-35.437, 44.8558) ccw
  line L468 (-35.7418, 44.8558) -> (-35.7418, 31.4192)
  arc A751 (-21.6956, 44.8558) -> (-22.0004, 45.1606) centre (-22.0004, 44.8558) ccw
  line L469 (-21.6956, 31.4192) -> (-21.6956, 44.8558)
  line L470 (-35.437, 31.1144) -> (-22.0004, 31.1144)
  line L471 (-35.7418, 31.1144) -> (-21.6956, 45.1606) construction
  line L472 (-21.6956, 31.1144) -> (-35.7418, 45.1606) construction
  arc A752 (-22.0004, 31.1144) -> (-21.6956, 31.4192) centre (-22.0004, 31.4192) ccw
  line L473 (-22.0004, 45.1606) -> (-35.437, 45.1606)
  arc A753 (-26.2168, 12.3692) -> (-25.912, 12.0644) centre (-25.912, 12.3692) ccw
  arc A754 (-25.912, 26.1106) -> (-26.2168, 25.8058) centre (-25.912, 25.8058) ccw
  line L474 (-26.2168, 25.8058) -> (-26.2168, 12.3692)
  arc A755 (-12.1706, 25.8058) -> (-12.4754, 26.1106) centre (-12.4754, 25.8058) ccw
  line L475 (-12.1706, 12.3692) -> (-12.1706, 25.8058)
  line L476 (-25.912, 12.0644) -> (-12.4754, 12.0644)
  line L477 (-26.2168, 12.0644) -> (-12.1706, 26.1106) construction
  line L478 (-12.1706, 12.0644) -> (-26.2168, 26.1106) construction
  arc A756 (-12.4754, 12.0644) -> (-12.1706, 12.3692) centre (-12.4754, 12.3692) ccw
  line L479 (-12.4754, 26.1106) -> (-25.912, 26.1106)
  arc A757 (-21.4543, -6.6808) -> (-21.1496, -6.9856) centre (-21.1496, -6.6808) ccw
  arc A758 (-21.1496, 7.0606) -> (-21.4543, 6.7558) centre (-21.1496, 6.7558) ccw
  line L480 (-21.4543, 6.7558) -> (-21.4543, -6.6808)
  arc A759 (-7.4081, 6.7558) -> (-7.713, 7.0606) centre (-7.713, 6.7558) ccw
  line L481 (-7.4081, -6.6808) -> (-7.4081, 6.7558)
  line L482 (-21.1496, -6.9856) -> (-7.713, -6.9856)
  line L483 (-21.4543, -6.9856) -> (-7.4081, 7.0606) construction
  line L484 (-7.4081, -6.9856) -> (-21.4543, 7.0606) construction
  arc A760 (-7.713, -6.9856) -> (-7.4081, -6.6808) centre (-7.713, -6.6808) ccw
  line L485 (-7.713, 7.0606) -> (-21.1496, 7.0606)
  arc A761 (-11.9293, -25.7308) -> (-11.6246, -26.0356) centre (-11.6246, -25.7308) ccw
  arc A762 (-11.6246, -11.9894) -> (-11.9293, -12.2942) centre (-11.6246, -12.2942) ccw
  line L486 (-11.9293, -12.2942) -> (-11.9293, -25.7308)
  arc A763 (2.1169, -12.2942) -> (1.812, -11.9894) centre (1.812, -12.2942) ccw
  line L487 (2.1169, -25.7308) -> (2.1169, -12.2942)
  line L488 (-11.6246, -26.0356) -> (1.812, -26.0356)
  line L489 (-11.9293, -26.0356) -> (2.1169, -11.9894) construction
  line L490 (2.1169, -26.0356) -> (-11.9293, -11.9894) construction
  arc A764 (1.812, -26.0356) -> (2.1169, -25.7308) centre (1.812, -25.7308) ccw
  line L491 (1.812, -11.9894) -> (-11.6246, -11.9894)
  arc A765 (-16.6918, 31.4192) -> (-16.3871, 31.1144) centre (-16.3871, 31.4192) ccw
  arc A766 (-16.3871, 45.1606) -> (-16.6918, 44.8558) centre (-16.3871, 44.8558) ccw
  line L492 (-16.6918, 44.8558) -> (-16.6918, 31.4192)
  arc A767 (-2.6456, 44.8558) -> (-2.9505, 45.1606) centre (-2.9505, 44.8558) ccw
  line L493 (-2.6456, 31.4192) -> (-2.6456, 44.8558)
  line L494 (-16.3871, 31.1144) -> (-2.9505, 31.1144)
  line L495 (-16.6918, 31.1144) -> (-2.6456, 45.1606) construction
  line L496 (-2.6456, 31.1144) -> (-16.6918, 45.1606) construction
  arc A768 (-2.9505, 31.1144) -> (-2.6456, 31.4192) centre (-2.9505, 31.4192) ccw
  line L497 (-2.9505, 45.1606) -> (-16.3871, 45.1606)
  arc A769 (-7.1668, 12.3692) -> (-6.8621, 12.0644) centre (-6.8621, 12.3692) ccw
  arc A770 (-6.8621, 26.1106) -> (-7.1668, 25.8058) centre (-6.8621, 25.8058) ccw
  line L498 (-7.1668, 25.8058) -> (-7.1668, 12.3692)
  arc A771 (6.8794, 25.8058) -> (6.5745, 26.1106) centre (6.5745, 25.8058) ccw
  line L499 (6.8794, 12.3692) -> (6.8794, 25.8058)
  line L500 (-6.8621, 12.0644) -> (6.5745, 12.0644)
  line L501 (-7.1668, 12.0644) -> (6.8794, 26.1106) construction
  line L502 (6.8794, 12.0644) -> (-7.1668, 26.1106) construction
  arc A772 (6.5745, 12.0644) -> (6.8794, 12.3692) centre (6.5745, 12.3692) ccw
  line L503 (6.5745, 26.1106) -> (-6.8621, 26.1106)
  arc A773 (-2.4043, -6.6808) -> (-2.0996, -6.9856) centre (-2.0996, -6.6808) ccw
  arc A774 (-2.0996, 7.0606) -> (-2.4043, 6.7558) centre (-2.0996, 6.7558) ccw
  line L504 (-2.4043, 6.7558) -> (-2.4043, -6.6808)
  arc A775 (11.6419, 6.7558) -> (11.337, 7.0606) centre (11.337, 6.7558) ccw
  line L505 (11.6419, -6.6808) -> (11.6419, 6.7558)
  line L506 (-2.0996, -6.9856) -> (11.337, -6.9856)
  line L507 (-2.4043, -6.9856) -> (11.6419, 7.0606) construction
  line L508 (11.6419, -6.9856) -> (-2.4043, 7.0606) construction
  arc A776 (11.337, -6.9856) -> (11.6419, -6.6808) centre (11.337, -6.6808) ccw
  line L509 (11.337, 7.0606) -> (-2.0996, 7.0606)
  arc A777 (7.1207, -25.7308) -> (7.4254, -26.0356) centre (7.4254, -25.7308) ccw
  arc A778 (7.4254, -11.9894) -> (7.1207, -12.2942) centre (7.4254, -12.2942) ccw
  line L510 (7.1207, -12.2942) -> (7.1207, -25.7308)
  arc A779 (21.1669, -12.2942) -> (20.862, -11.9894) centre (20.862, -12.2942) ccw
  line L511 (21.1669, -25.7308) -> (21.1669, -12.2942)
  line L512 (7.4254, -26.0356) -> (20.862, -26.0356)
  line L513 (7.1207, -26.0356) -> (21.1669, -11.9894) construction
  line L514 (21.1669, -26.0356) -> (7.1207, -11.9894) construction
  arc A780 (20.862, -26.0356) -> (21.1669, -25.7308) centre (20.862, -25.7308) ccw
  line L515 (20.862, -11.9894) -> (7.4254, -11.9894)
  arc A781 (2.3582, 31.4192) -> (2.6629, 31.1144) centre (2.6629, 31.4192) ccw
  arc A782 (2.6629, 45.1606) -> (2.3582, 44.8558) centre (2.6629, 44.8558) ccw
  line L516 (2.3582, 44.8558) -> (2.3582, 31.4192)
  arc A783 (16.4044, 44.8558) -> (16.0995, 45.1606) centre (16.0995, 44.8558) ccw
  line L517 (16.4044, 31.4192) -> (16.4044, 44.8558)
  line L518 (2.6629, 31.1144) -> (16.0995, 31.1144)
  line L519 (2.3582, 31.1144) -> (16.4044, 45.1606) construction
  line L520 (16.4044, 31.1144) -> (2.3582, 45.1606) construction
  arc A784 (16.0995, 31.1144) -> (16.4044, 31.4192) centre (16.0995, 31.4192) ccw
  line L521 (16.0995, 45.1606) -> (2.6629, 45.1606)
  arc A785 (11.8832, 12.3692) -> (12.188, 12.0644) centre (12.188, 12.3692) ccw
  arc A786 (12.188, 26.1106) -> (11.8832, 25.8058) centre (12.188, 25.8058) ccw
  line L522 (11.8832, 25.8058) -> (11.8832, 12.3692)
  arc A787 (25.9294, 25.8058) -> (25.6245, 26.1106) centre (25.6245, 25.8058) ccw
  line L523 (25.9294, 12.3692) -> (25.9294, 25.8058)
  line L524 (12.188, 12.0644) -> (25.6245, 12.0644)
  line L525 (11.8832, 12.0644) -> (25.9294, 26.1106) construction
  line L526 (25.9294, 12.0644) -> (11.8832, 26.1106) construction
  arc A788 (25.6245, 12.0644) -> (25.9294, 12.3692) centre (25.6245, 12.3692) ccw
  line L527 (25.6245, 26.1106) -> (12.188, 26.1106)
  arc A789 (16.6457, -6.6808) -> (16.9505, -6.9856) centre (16.9505, -6.6808) ccw
  arc A790 (16.9505, 7.0606) -> (16.6457, 6.7558) centre (16.9505, 6.7558) ccw
  line L528 (16.6457, 6.7558) -> (16.6457, -6.6808)
  arc A791 (30.6919, 6.7558) -> (30.3871, 7.0606) centre (30.3871, 6.7558) ccw
  line L529 (30.6919, -6.6808) -> (30.6919, 6.7558)
  line L530 (16.9505, -6.9856) -> (30.3871, -6.9856)
  line L531 (16.6457, -6.9856) -> (30.6919, 7.0606) construction
  line L532 (30.6919, -6.9856) -> (16.6457, 7.0606) construction
  arc A792 (30.3871, -6.9856) -> (30.6919, -6.6808) centre (30.3871, -6.6808) ccw
  line L533 (30.3871, 7.0606) -> (16.9505, 7.0606)
  arc A793 (26.1707, -25.7308) -> (26.4755, -26.0356) centre (26.4755, -25.7308) ccw
  arc A794 (26.4755, -11.9894) -> (26.1707, -12.2942) centre (26.4755, -12.2942) ccw
  line L534 (26.1707, -12.2942) -> (26.1707, -25.7308)
  arc A795 (40.2169, -12.2942) -> (39.9121, -11.9894) centre (39.9121, -12.2942) ccw
  line L535 (40.2169, -25.7308) -> (40.2169, -12.2942)
  line L536 (26.4755, -26.0356) -> (39.9121, -26.0356)
  line L537 (26.1707, -26.0356) -> (40.2169, -11.9894) construction
  line L538 (40.2169, -26.0356) -> (26.1707, -11.9894) construction
  arc A796 (39.9121, -26.0356) -> (40.2169, -25.7308) centre (39.9121, -25.7308) ccw
  line L539 (39.9121, -11.9894) -> (26.4755, -11.9894)
  arc A797 (21.4082, 31.4192) -> (21.713, 31.1144) centre (21.713, 31.4192) ccw
  arc A798 (21.713, 45.1606) -> (21.4082, 44.8558) centre (21.713, 44.8558) ccw
  line L540 (21.4082, 44.8558) -> (21.4082, 31.4192)
  arc A799 (35.4544, 44.8558) -> (35.1496, 45.1606) centre (35.1496, 44.8558) ccw
  line L541 (35.4544, 31.4192) -> (35.4544, 44.8558)
  line L542 (21.713, 31.1144) -> (35.1496, 31.1144)
  line L543 (21.4082, 31.1144) -> (35.4544, 45.1606) construction
  line L544 (35.4544, 31.1144) -> (21.4082, 45.1606) construction
  arc A800 (35.1496, 31.1144) -> (35.4544, 31.4192) centre (35.1496, 31.4192) ccw
  line L545 (35.1496, 45.1606) -> (21.713, 45.1606)
  arc A801 (30.9332, 12.3692) -> (31.238, 12.0644) centre (31.238, 12.3692) ccw
  arc A802 (31.238, 26.1106) -> (30.9332, 25.8058) centre (31.238, 25.8058) ccw
  line L546 (30.9332, 25.8058) -> (30.9332, 12.3692)
  arc A803 (44.9794, 25.8058) -> (44.6746, 26.1106) centre (44.6746, 25.8058) ccw
  line L547 (44.9794, 12.3692) -> (44.9794, 25.8058)
  line L548 (31.238, 12.0644) -> (44.6746, 12.0644)
  line L549 (30.9332, 12.0644) -> (44.9794, 26.1106) construction
  line L550 (44.9794, 12.0644) -> (30.9332, 26.1106) construction
  arc A804 (44.6746, 12.0644) -> (44.9794, 12.3692) centre (44.6746, 12.3692) ccw
  line L551 (44.6746, 26.1106) -> (31.238, 26.1106)
  arc A805 (35.6957, -6.6808) -> (36.0005, -6.9856) centre (36.0005, -6.6808) ccw
  arc A806 (36.0005, 7.0606) -> (35.6957, 6.7558) centre (36.0005, 6.7558) ccw
  line L552 (35.6957, 6.7558) -> (35.6957, -6.6808)
  arc A807 (49.7419, 6.7558) -> (49.4371, 7.0606) centre (49.4371, 6.7558) ccw
  line L553 (49.7419, -6.6808) -> (49.7419, 6.7558)
  line L554 (36.0005, -6.9856) -> (49.4371, -6.9856)
  line L555 (35.6957, -6.9856) -> (49.7419, 7.0606) construction
  line L556 (49.7419, -6.9856) -> (35.6957, 7.0606) construction
  arc A808 (49.4371, -6.9856) -> (49.7419, -6.6808) centre (49.4371, -6.6808) ccw
  line L557 (49.4371, 7.0606) -> (36.0005, 7.0606)
  arc A809 (45.2207, -25.7308) -> (45.5255, -26.0356) centre (45.5255, -25.7308) ccw
  arc A810 (45.5255, -11.9894) -> (45.2207, -12.2942) centre (45.5255, -12.2942) ccw
  line L558 (45.2207, -12.2942) -> (45.2207, -25.7308)
  arc A811 (59.2669, -12.2942) -> (58.9621, -11.9894) centre (58.9621, -12.2942) ccw
  line L559 (59.2669, -25.7308) -> (59.2669, -12.2942)
  line L560 (45.5255, -26.0356) -> (58.9621, -26.0356)
  line L561 (45.2207, -26.0356) -> (59.2669, -11.9894) construction
  line L562 (59.2669, -26.0356) -> (45.2207, -11.9894) construction
  arc A812 (58.9621, -26.0356) -> (59.2669, -25.7308) centre (58.9621, -25.7308) ccw
  line L563 (58.9621, -11.9894) -> (45.5255, -11.9894)
  arc A813 (40.4582, 31.4192) -> (40.763, 31.1144) centre (40.763, 31.4192) ccw
  arc A814 (40.763, 45.1606) -> (40.4582, 44.8558) centre (40.763, 44.8558) ccw
  line L564 (40.4582, 44.8558) -> (40.4582, 31.4192)
  arc A815 (54.5044, 44.8558) -> (54.1996, 45.1606) centre (54.1996, 44.8558) ccw
  line L565 (54.5044, 31.4192) -> (54.5044, 44.8558)
  line L566 (40.763, 31.1144) -> (54.1996, 31.1144)
  line L567 (40.4582, 31.1144) -> (54.5044, 45.1606) construction
  line L568 (54.5044, 31.1144) -> (40.4582, 45.1606) construction
  arc A816 (54.1996, 31.1144) -> (54.5044, 31.4192) centre (54.1996, 31.4192) ccw
  line L569 (54.1996, 45.1606) -> (40.763, 45.1606)
  arc A817 (59.5082, 31.4192) -> (59.8129, 31.1144) centre (59.8129, 31.4192) ccw
  arc A818 (59.8129, 45.1606) -> (59.5082, 44.8558) centre (59.8129, 44.8558) ccw
  line L570 (59.5082, 44.8558) -> (59.5082, 31.4192)
  arc A819 (73.5544, 44.8558) -> (73.2495, 45.1606) centre (73.2495, 44.8558) ccw
  line L571 (73.5544, 31.4192) -> (73.5544, 44.8558)
  line L572 (59.8129, 31.1144) -> (73.2495, 31.1144)
  line L573 (59.5082, 31.1144) -> (73.5544, 45.1606) construction
  line L574 (73.5544, 31.1144) -> (59.5082, 45.1606) construction
  arc A820 (73.2495, 31.1144) -> (73.5544, 31.4192) centre (73.2495, 31.4192) ccw
  line L575 (73.2495, 45.1606) -> (59.8129, 45.1606)
  arc A821 (49.9832, 12.3692) -> (50.288, 12.0644) centre (50.288, 12.3692) ccw
  arc A822 (50.288, 26.1106) -> (49.9832, 25.8058) centre (50.288, 25.8058) ccw
  line L576 (49.9832, 25.8058) -> (49.9832, 12.3692)
  arc A823 (64.0294, 25.8058) -> (63.7246, 26.1106) centre (63.7246, 25.8058) ccw
  line L577 (64.0294, 12.3692) -> (64.0294, 25.8058)
  line L578 (50.288, 12.0644) -> (63.7246, 12.0644)
  line L579 (49.9832, 12.0644) -> (64.0294, 26.1106) construction
  line L580 (64.0294, 12.0644) -> (49.9832, 26.1106) construction
  arc A824 (63.7246, 12.0644) -> (64.0294, 12.3692) centre (63.7246, 12.3692) ccw
  line L581 (63.7246, 26.1106) -> (50.288, 26.1106)
  arc A825 (69.0332, 12.3692) -> (69.338, 12.0644) centre (69.338, 12.3692) ccw
  arc A826 (69.338, 26.1106) -> (69.0332, 25.8058) centre (69.338, 25.8058) ccw
  line L582 (69.0332, 25.8058) -> (69.0332, 12.3692)
  arc A827 (83.0794, 25.8058) -> (82.7746, 26.1106) centre (82.7746, 25.8058) ccw
  line L583 (83.0794, 12.3692) -> (83.0794, 25.8058)
  line L584 (69.338, 12.0644) -> (82.7746, 12.0644)
  line L585 (69.0332, 12.0644) -> (83.0794, 26.1106) construction
  line L586 (83.0794, 12.0644) -> (69.0332, 26.1106) construction
  arc A828 (82.7746, 12.0644) -> (83.0794, 12.3692) centre (82.7746, 12.3692) ccw
  line L587 (82.7746, 26.1106) -> (69.338, 26.1106)
  arc A829 (54.7457, -6.6808) -> (55.0504, -6.9856) centre (55.0504, -6.6808) ccw
  arc A830 (55.0504, 7.0606) -> (54.7457, 6.7558) centre (55.0504, 6.7558) ccw
  line L588 (54.7457, 6.7558) -> (54.7457, -6.6808)
  arc A831 (68.7919, 6.7558) -> (68.487, 7.0606) centre (68.487, 6.7558) ccw
  line L589 (68.7919, -6.6808) -> (68.7919, 6.7558)
  line L590 (55.0504, -6.9856) -> (68.487, -6.9856)
  line L591 (54.7457, -6.9856) -> (68.7919, 7.0606) construction
  line L592 (68.7919, -6.9856) -> (54.7457, 7.0606) construction
  arc A832 (68.487, -6.9856) -> (68.7919, -6.6808) centre (68.487, -6.6808) ccw
  line L593 (68.487, 7.0606) -> (55.0504, 7.0606)
  arc A833 (73.7957, -6.6808) -> (74.1004, -6.9856) centre (74.1004, -6.6808) ccw
  arc A834 (74.1004, 7.0606) -> (73.7957, 6.7558) centre (74.1004, 6.7558) ccw
  line L594 (73.7957, 6.7558) -> (73.7957, -6.6808)
  arc A835 (87.8419, 6.7558) -> (87.537, 7.0606) centre (87.537, 6.7558) ccw
  line L595 (87.8419, -6.6808) -> (87.8419, 6.7558)
  line L596 (74.1004, -6.9856) -> (87.537, -6.9856)
  line L597 (73.7957, -6.9856) -> (87.8419, 7.0606) construction
  line L598 (87.8419, -6.9856) -> (73.7957, 7.0606) construction
  arc A836 (87.537, -6.9856) -> (87.8419, -6.6808) centre (87.537, -6.6808) ccw
  line L599 (87.537, 7.0606) -> (74.1004, 7.0606)
  arc A837 (64.2707, -25.7308) -> (64.5754, -26.0356) centre (64.5754, -25.7308) ccw
  arc A838 (64.5754, -11.9894) -> (64.2707, -12.2942) centre (64.5754, -12.2942) ccw
  line L600 (64.2707, -12.2942) -> (64.2707, -25.7308)
  arc A839 (78.3169, -12.2942) -> (78.012, -11.9894) centre (78.012, -12.2942) ccw
  line L601 (78.3169, -25.7308) -> (78.3169, -12.2942)
  line L602 (64.5754, -26.0356) -> (78.012, -26.0356)
  line L603 (64.2707, -26.0356) -> (78.3169, -11.9894) construction
  line L604 (78.3169, -26.0356) -> (64.2707, -11.9894) construction
  arc A840 (78.012, -26.0356) -> (78.3169, -25.7308) centre (78.012, -25.7308) ccw
  line L605 (78.012, -11.9894) -> (64.5754, -11.9894)
  arc A841 (40.4582, -44.7808) -> (40.763, -45.0856) centre (40.763, -44.7808) ccw
  arc A842 (40.763, -31.0394) -> (40.4582, -31.3442) centre (40.763, -31.3442) ccw
  line L606 (40.4582, -31.3442) -> (40.4582, -44.7808)
  arc A843 (54.5044, -31.3442) -> (54.1996, -31.0394) centre (54.1996, -31.3442) ccw
  line L607 (54.5044, -44.7808) -> (54.5044, -31.3442)
  line L608 (40.763, -45.0856) -> (54.1996, -45.0856)
  line L609 (40.4582, -45.0856) -> (54.5044, -31.0394) construction
  line L610 (54.5044, -45.0856) -> (40.4582, -31.0394) construction
  arc A844 (54.1996, -45.0856) -> (54.5044, -44.7808) centre (54.1996, -44.7808) ccw
  line L611 (54.1996, -31.0394) -> (40.763, -31.0394)
  arc A845 (59.5082, -44.7808) -> (59.8129, -45.0856) centre (59.8129, -44.7808) ccw
  arc A846 (59.8129, -31.0394) -> (59.5082, -31.3442) centre (59.8129, -31.3442) ccw
  line L612 (59.5082, -31.3442) -> (59.5082, -44.7808)
  arc A847 (73.5544, -31.3442) -> (73.2495, -31.0394) centre (73.2495, -31.3442) ccw
  line L613 (73.5544, -44.7808) -> (73.5544, -31.3442)
  line L614 (59.8129, -45.0856) -> (73.2495, -45.0856)
  line L615 (59.5082, -45.0856) -> (73.5544, -31.0394) construction
  line L616 (73.5544, -45.0856) -> (59.5082, -31.0394) construction
  arc A848 (73.2495, -45.0856) -> (73.5544, -44.7808) centre (73.2495, -44.7808) ccw
  line L617 (73.2495, -31.0394) -> (59.8129, -31.0394)
  arc A849 (78.5582, -44.7808) -> (78.863, -45.0856) centre (78.863, -44.7808) ccw
  arc A850 (78.863, -31.0394) -> (78.5582, -31.3442) centre (78.863, -31.3442) ccw
  line L618 (78.5582, -31.3442) -> (78.5582, -44.7808)
  arc A851 (92.6044, -31.3442) -> (92.2996, -31.0394) centre (92.2996, -31.3442) ccw
  line L619 (92.6044, -44.7808) -> (92.6044, -31.3442)
  line L620 (78.863, -45.0856) -> (92.2996, -45.0856)
  line L621 (78.5582, -45.0856) -> (92.6044, -31.0394) construction
  line L622 (92.6044, -45.0856) -> (78.5582, -31.0394) construction
  arc A852 (92.2996, -45.0856) -> (92.6044, -44.7808) centre (92.2996, -44.7808) ccw
  line L623 (92.2996, -31.0394) -> (78.863, -31.0394)
  arc A853 (97.6082, -44.7808) -> (97.9129, -45.0856) centre (97.9129, -44.7808) ccw
  arc A854 (97.9129, -31.0394) -> (97.6082, -31.3442) centre (97.9129, -31.3442) ccw
  line L624 (97.6082, -31.3442) -> (97.6082, -44.7808)
  arc A855 (111.6544, -31.3442) -> (111.3495, -31.0394) centre (111.3495, -31.3442) ccw
  line L625 (111.6544, -44.7808) -> (111.6544, -31.3442)
  line L626 (97.9129, -45.0856) -> (111.3495, -45.0856)
  line L627 (97.6082, -45.0856) -> (111.6544, -31.0394) construction
  line L628 (111.6544, -45.0856) -> (97.6082, -31.0394) construction
  arc A856 (111.3495, -45.0856) -> (111.6544, -44.7808) centre (111.3495, -44.7808) ccw
  line L629 (111.3495, -31.0394) -> (97.9129, -31.0394)
  arc A857 (116.6582, -44.7808) -> (116.9629, -45.0856) centre (116.9629, -44.7808) ccw
  arc A858 (116.9629, -31.0394) -> (116.6582, -31.3442) centre (116.9629, -31.3442) ccw
  line L630 (116.6582, -31.3442) -> (116.6582, -44.7808)
  arc A859 (130.7044, -31.3442) -> (130.3995, -31.0394) centre (130.3995, -31.3442) ccw
  line L631 (130.7044, -44.7808) -> (130.7044, -31.3442)
  line L632 (116.9629, -45.0856) -> (130.3995, -45.0856)
  line L633 (116.6582, -45.0856) -> (130.7044, -31.0394) construction
  line L634 (130.7044, -45.0856) -> (116.6582, -31.0394) construction
  arc A860 (130.3995, -45.0856) -> (130.7044, -44.7808) centre (130.3995, -44.7808) ccw
  line L635 (130.3995, -31.0394) -> (116.9629, -31.0394)
  arc A861 (135.7082, -44.7808) -> (136.0129, -45.0856) centre (136.0129, -44.7808) ccw
  arc A862 (136.0129, -31.0394) -> (135.7082, -31.3442) centre (136.0129, -31.3442) ccw
  line L636 (135.7082, -31.3442) -> (135.7082, -44.7808)
  arc A863 (149.7544, -31.3442) -> (149.4495, -31.0394) centre (149.4495, -31.3442) ccw
  line L637 (149.7544, -44.7808) -> (149.7544, -31.3442)
  line L638 (136.0129, -45.0856) -> (149.4495, -45.0856)
  line L639 (135.7082, -45.0856) -> (149.7544, -31.0394) construction
  line L640 (149.7544, -45.0856) -> (135.7082, -31.0394) construction
  arc A864 (149.4495, -45.0856) -> (149.7544, -44.7808) centre (149.4495, -44.7808) ccw
  line L641 (149.4495, -31.0394) -> (136.0129, -31.0394)
  arc A865 (135.7082, -25.7308) -> (136.0129, -26.0356) centre (136.0129, -25.7308) ccw
  arc A866 (136.0129, -11.9894) -> (135.7082, -12.2942) centre (136.0129, -12.2942) ccw
  line L642 (135.7082, -12.2942) -> (135.7082, -25.7308)
  arc A867 (149.7544, -12.2942) -> (149.4495, -11.9894) centre (149.4495, -12.2942) ccw
  line L643 (149.7544, -25.7308) -> (149.7544, -12.2942)
  line L644 (136.0129, -26.0356) -> (149.4495, -26.0356)
  line L645 (135.7082, -26.0356) -> (149.7544, -11.9894) construction
  line L646 (149.7544, -26.0356) -> (135.7082, -11.9894) construction
  arc A868 (149.4495, -26.0356) -> (149.7544, -25.7308) centre (149.4495, -25.7308) ccw
  line L647 (149.4495, -11.9894) -> (136.0129, -11.9894)
  arc A869 (116.6582, -25.7308) -> (116.9629, -26.0356) centre (116.9629, -25.7308) ccw
  arc A870 (116.9629, -11.9894) -> (116.6582, -12.2942) centre (116.9629, -12.2942) ccw
  line L648 (116.6582, -12.2942) -> (116.6582, -25.7308)
  arc A871 (130.7044, -12.2942) -> (130.3995, -11.9894) centre (130.3995, -12.2942) ccw
  line L649 (130.7044, -25.7308) -> (130.7044, -12.2942)
  line L650 (116.9629, -26.0356) -> (130.3995, -26.0356)
  line L651 (116.6582, -26.0356) -> (130.7044, -11.9894) construction
  line L652 (130.7044, -26.0356) -> (116.6582, -11.9894) construction